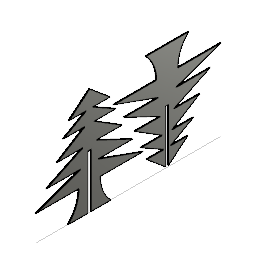
Tree v1 (Autodesk Fusion 360 design; units mm, degrees)
Autodesk Fusion 360 part; units mm, degrees
sketch "Sketch1" plane through (0, 0, 0) normal (1, 0, 0) x (0, 0, -1)
  line L0 (0, 0) -> (140, 0)
  line L1 (140, 0) -> (140, 140)
  line L2 (140, 140) -> (0, 140)
  line L3 (0, 140) -> (0, 0)
  line L4 (70, 0) -> (95, 0)
  line L5 (70, 0) -> (45, 0)
  line L6 (57.5, 0) -> (82.5, 0)
  arc A0 (45, 0) -> (57.5, 30) centre (15.25, 30) ccw
  arc A1 (82.5, 30) -> (95, 0) centre (124.75, 30) ccw
  line L7 (57.5, 30) -> (7.5, 30)
  line L8 (7.5, 30) -> (11.6123, 30)
  line L9 (7.5, 30) -> (59.6212, 48.6667)
  line L10 (59.6212, 48.6667) -> (19.6212, 48.6667)
  line L11 (19.6212, 48.6667) -> (61.9142, 68.8448)
  line L12 (61.9142, 68.8448) -> (31.9142, 68.8448)
  line L13 (31.9142, 68.8448) -> (64.1928, 88.8963)
  line L14 (64.1928, 88.8963) -> (39.1928, 88.8963)
  line L15 (39.1928, 88.8963) -> (65.9101, 104.0086)
  line L16 (65.9101, 104.0086) -> (45.9101, 104.0086)
  line L17 (45.9101, 104.0086) -> (68.0131, 122.5152)
  line L18 (82.5, 30) -> (132.5, 30)
  line L19 (132.5, 30) -> (80.3788, 48.6667)
  line L20 (80.3788, 48.6667) -> (120.3788, 48.6667)
  line L21 (120.3788, 48.6667) -> (78.0858, 68.8448)
  line L22 (78.0858, 68.8448) -> (108.0858, 68.8448)
  line L23 (108.0858, 68.8448) -> (75.8072, 88.8963)
  line L24 (75.8072, 88.8963) -> (100.8072, 88.8963)
  line L25 (100.8072, 88.8963) -> (74.0899, 104.0086)
  line L26 (74.0899, 104.0086) -> (94.0899, 104.0086)
  line L27 (94.0899, 104.0086) -> (71.9869, 122.5152)
  line L28 (71.9869, 122.5152) -> (70.1135, 124.2739)
  line L29 (70.1135, 124.2739) -> (68.0131, 122.5152)
  dimension "d1" = 140
  dimension "d2" = 140
  dimension "d7" = 40
  dimension "d8" = 30
  dimension "d10" = 25
  dimension "d11" = 20
  dimension "d13" = 50
  dimension "d14" = 40
  dimension "d15" = 30
  dimension "d16" = 25
  dimension "d17" = 20
  constraint horizontal L0
  constraint vertical L1
  constraint horizontal L2
  constraint vertical L3
  constraint coincident L0.start L3.end
  constraint midpoint L0 L4.start
  constraint horizontal L6
  constraint midpoint L5 L6.start
  constraint coincident L7 L8.end
  constraint horizontal L14
  constraint parallel L17 L29
  measures "d1" distance of L0.start L0.end
  measures "d2" distance of L0.start L2.end
  measures "d7" distance of L9.end L10.end
  measures "d8" distance of L11.end L12.end
  measures "d10" distance of L13.end L14.end
  measures "d11" distance of L15.end L16.end
  measures "d13" distance of A1.start L18.end
  measures "d14" distance of L19.end L20.end
  measures "d15" distance of L21.end L22.end
  measures "d16" distance of L23.end L24.end
  measures "d17" distance of L25.end L26.end
extrude "Extrude1" add sketch "Sketch1" along normal blind 1 contours L0 L4 L5 L6 A0 A1 L7 L8 L9 L10 L11 L12 L13 L14 L15 L16 L17 L18 L19 L20 L21 L22 L23 L24 L25 L26 L27 L28 L29 makes body 1
copy_body "CopyPasteBodies1" bodies 1 makes body 2
move_body "Move1" bodies 2 to x (1, 0, 0) y (0, -1, 0) z (0, 0, -1) at (0, 124.2739, -230)
sketch "Sketch2" plane through (1, 0, 0) normal (1, 0, 0) x (0, 0, -1)
  line L0 (82.5, 30) -> (132.5, 30)
  line L1 (132.5, 30) -> (80.3788, 48.6667)
  line L2 (80.3788, 48.6667) -> (120.3788, 48.6667)
  line L3 (120.3788, 48.6667) -> (78.0858, 68.8448)
  line L4 (78.0858, 68.8448) -> (108.0858, 68.8448)
  line L5 (108.0858, 68.8448) -> (75.8072, 88.8963)
  line L6 (75.8072, 88.8963) -> (100.8072, 88.8963)
  line L7 (100.8072, 88.8963) -> (74.0899, 104.0086)
  line L8 (74.0899, 104.0086) -> (94.0899, 104.0086)
  line L9 (94.0899, 104.0086) -> (71.9869, 122.5152)
  line L10 (71.9869, 122.5152) -> (70.1135, 124.2739)
  line L11 (70.1135, 124.2739) -> (45.9101, 104.0086)
  line L12 (45.9101, 104.0086) -> (65.9101, 104.0086)
  line L13 (65.9101, 104.0086) -> (39.1928, 88.8963)
  line L14 (39.1928, 88.8963) -> (64.1928, 88.8963)
  line L15 (64.1928, 88.8963) -> (31.9142, 68.8448)
  line L16 (31.9142, 68.8448) -> (61.9142, 68.8448)
  line L17 (61.9142, 68.8448) -> (19.6212, 48.6667)
  line L18 (19.6212, 48.6667) -> (59.6212, 48.6667)
  line L19 (59.6212, 48.6667) -> (7.5, 30)
  line L20 (7.5, 30) -> (57.5, 30)
  arc A0 (45, 0) -> (57.5, 30) centre (15.25, 30) ccw
  line L21 (45, 0) -> (95, 0)
  arc A1 (82.5, 30) -> (95, 0) centre (124.75, 30) ccw
  line L22 (159.8865, 0) -> (161.3865, 0)
  line L23 (161.3865, 0) -> (158.3865, 0)
  line L24 (158.3865, 0) -> (158.3865, 62.5)
  line L25 (158.3865, 62.5) -> (161.3865, 62.5)
  line L26 (161.3865, 62.5) -> (161.3865, 0)
  point P0 (159.8865, 0)
  dimension "d21" = 1.5
  dimension "d22" = 62.5
  dimension "d23" = 3
  constraint coincident P0 L22.start
  constraint horizontal L22
  constraint horizontal L23
  constraint vertical L24
  constraint horizontal L25
  constraint vertical L26
  measures "d21" distance of P0 L22.end
  measures "d22" distance of L22.end L25.end
  measures "d23" distance of L22.end L23.end
extrude "Extrude2" cut sketch "Sketch2" against normal blind 1 contours L22 L23 L24 L25 L26 bodies 2
sketch "Sketch3" plane through (1, 0, 0) normal (1, 0, 0) x (0, 0, -1)
  line L0 (82.5, 30) -> (132.5, 30)
  line L1 (132.5, 30) -> (80.3788, 48.6667)
  line L2 (80.3788, 48.6667) -> (120.3788, 48.6667)
  line L3 (120.3788, 48.6667) -> (78.0858, 68.8448)
  line L4 (78.0858, 68.8448) -> (108.0858, 68.8448)
  line L5 (108.0858, 68.8448) -> (75.8072, 88.8963)
  line L6 (75.8072, 88.8963) -> (100.8072, 88.8963)
  line L7 (100.8072, 88.8963) -> (74.0899, 104.0086)
  line L8 (74.0899, 104.0086) -> (94.0899, 104.0086)
  line L9 (94.0899, 104.0086) -> (71.9869, 122.5152)
  line L10 (71.9869, 122.5152) -> (70.1135, 124.2739)
  line L11 (70.1135, 124.2739) -> (45.9101, 104.0086)
  line L12 (45.9101, 104.0086) -> (65.9101, 104.0086)
  line L13 (65.9101, 104.0086) -> (39.1928, 88.8963)
  line L14 (39.1928, 88.8963) -> (64.1928, 88.8963)
  line L15 (64.1928, 88.8963) -> (31.9142, 68.8448)
  line L16 (31.9142, 68.8448) -> (61.9142, 68.8448)
  line L17 (61.9142, 68.8448) -> (19.6212, 48.6667)
  line L18 (19.6212, 48.6667) -> (59.6212, 48.6667)
  line L19 (59.6212, 48.6667) -> (7.5, 30)
  line L20 (7.5, 30) -> (57.5, 30)
  arc A0 (45, 0) -> (57.5, 30) centre (15.25, 30) ccw
  line L21 (45, 0) -> (95, 0)
  arc A1 (82.5, 30) -> (95, 0) centre (124.75, 30) ccw
  line L22 (70, 0) -> (71.75, 0)
  line L23 (71.75, 0) -> (68.25, 0)
  line L24 (68.25, 0) -> (68.25, 62.5)
  line L25 (68.25, 62.5) -> (71.75, 62.5)
  line L26 (71.75, 62.5) -> (71.75, 0)
  dimension "d26" = 1.75
  dimension "d27" = 62.5
  dimension "d28" = 3.5
  constraint midpoint L21 L22.start
  constraint horizontal L22
  constraint horizontal L23
  constraint vertical L24
  constraint horizontal L25
  constraint vertical L26
  measures "d26" distance of L22.start L22.end
  measures "d27" distance of L22.end L25.end
  measures "d28" distance of L22.end L23.end
extrude "Extrude3" cut sketch "Sketch3" against normal blind 1 contours L21 L22 L23 L24 L25 L26 bodies 1
